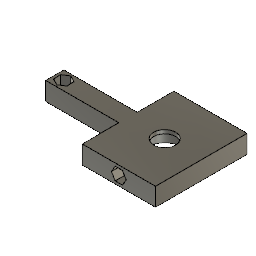
Hub Adapter (Autodesk Fusion 360 design; units mm, degrees)
Autodesk Fusion 360 part; units mm, degrees
sketch "Top" plane through (0, 0, 0) normal (0, 0, 1) x (1, 0, 0)
  line L0 (0, 0) -> (40, 0)
  line L1 (40, 0) -> (40, 50)
  line L2 (40, 50) -> (0, 50)
  line L3 (0, 50) -> (0, 0)
  circle A0 centre (20, 25) radius 11.2
  circle A1 centre (20, 25) radius 6
  dimension "d6" = 40
  dimension "d7" = 50
  dimension "d11" = 22.4
  dimension "d12" = 25
  dimension "d13" = 20
  dimension "d27" = 12
  constraint horizontal L0
  constraint vertical L1
  constraint horizontal L2
  constraint vertical L3
  constraint coincident L0.start L3.end
  constraint concentric A0 A1
  measures "d6" distance of L0.start L0.end
  measures "d7" distance of L0.start L2.end
  measures "d11" diameter of A0
  measures "d12" distance of L2 A0.centre
  measures "d13" distance of L1 A0.centre
  measures "d27" diameter of A1
extrude "Extrude1" add sketch "Top" along normal blind 10 contours L0 L1 L2 L3 | A0 | A1
extrude "Extrude2" cut sketch "Top" along normal blind 8 contours A0 | A1
extrude "Extrude5" cut sketch "Top" along normal blind 110 contours A1
sketch "Sketch3" plane through (0, 0, 0) normal (0, -1, 0) x (1, 0, 0)
  line L0 (0, 0) -> (40, 0)
  line L1 (40, 0) -> (40, 10)
  line L2 (40, 10) -> (0, 10)
  line L3 (0, 10) -> (0, 0)
  line L4 (24, 5) -> (22, 8.4641)
  line L5 (22, 8.4641) -> (18, 8.4641)
  line L6 (18, 8.4641) -> (16, 5)
  line L7 (16, 5) -> (18, 1.5359)
  line L8 (18, 1.5359) -> (22, 1.5359)
  line L9 (22, 1.5359) -> (24, 5)
  point P0 (20, 5)
  dimension "d34" = 4
  dimension "d37" = 20
  dimension "d38" = 5
  measures "d34" distance of L4.start P0
  measures "d37" distance of L3 P0
  measures "d38" distance of L2 P0
extrude "Extrude6" cut sketch "Sketch3" against normal blind 5 contours L4 L5 L6 L7 L8 L9
sketch "Sketch4" plane through (0, 50, 0) normal (0, 1, 0) x (-1, 0, 0)
  line L0 (-40, 0) -> (0, 0)
  line L1 (0, 0) -> (0, 10)
  line L2 (0, 10) -> (-40, 10)
  line L3 (-40, 10) -> (-40, 0)
  line L4 (-22.8284, 7.8284) -> (-23.8637, 3.9647)
  line L5 (-23.8637, 3.9647) -> (-21.0353, 1.1363)
  line L6 (-21.0353, 1.1363) -> (-17.1716, 2.1716)
  line L7 (-17.1716, 2.1716) -> (-16.1363, 6.0353)
  line L8 (-16.1363, 6.0353) -> (-18.9647, 8.8637)
  line L9 (-18.9647, 8.8637) -> (-22.8284, 7.8284)
  point P0 (-20, 5)
  dimension "d39" = 4
  dimension "d42" = 20
  dimension "d43" = 5
  measures "d39" distance of L4.start P0
  measures "d42" distance of L3 P0
  measures "d43" distance of L2 P0
extrude "Extrude7" cut sketch "Sketch4" against normal blind 5 contours L4 L5 L6 L7 L8 L9
sketch "Sketch5" plane through (0, 0, 0) normal (-1, 0, 0) x (0, -1, 0)
  line L0 (-50, 0) -> (0, 0)
  line L1 (0, 0) -> (0, 10)
  line L2 (0, 10) -> (-50, 10)
  line L3 (-50, 10) -> (-50, 0)
  line L4 (-30, 10) -> (-20, 10)
  line L5 (-20, 10) -> (-20, 0)
  line L6 (-20, 0) -> (-30, 0)
  line L7 (-30, 0) -> (-30, 10)
  dimension "d50" = 10
  dimension "d51" = 10
  dimension "d52" = 20
  constraint horizontal L4
  constraint vertical L5
  constraint horizontal L6
  constraint vertical L7
  constraint coincident L2 L4.start
  measures "d50" distance of L4.start L4.end
  measures "d51" distance of L4.start L6.end
  measures "d52" distance of L3 L7
extrude "Extrude8" add sketch "Sketch5" along normal blind 40 contours L0 L2 L4 L5 L6 L7
sketch "Sketch6" plane through (0, 0, 0) normal (0, 0, -1) x (1, 0, 0)
  circle A0 centre (20, -25) radius 11.2
  line L0 (0, -30) -> (0, -50)
  line L1 (0, -50) -> (40, -50)
  line L2 (40, -50) -> (40, 0)
  line L3 (40, 0) -> (0, 0)
  line L4 (0, 0) -> (0, -20)
  line L5 (0, -20) -> (-40, -20)
  line L6 (-40, -20) -> (-40, -30)
  line L7 (-40, -30) -> (0, -30)
  line L8 (-31.6559, -27.1948) -> (-31.4272, -23.2013)
  line L9 (-31.4272, -23.2013) -> (-34.7713, -21.0065)
  line L10 (-34.7713, -21.0065) -> (-38.3441, -22.8052)
  line L11 (-38.3441, -22.8052) -> (-38.5728, -26.7987)
  line L12 (-38.5728, -26.7987) -> (-35.2287, -28.9935)
  line L13 (-35.2287, -28.9935) -> (-31.6559, -27.1948)
  point P0 (-35, -25)
  dimension "d55" = 4
  dimension "d56" = 5
  dimension "d57" = 5
  measures "d55" distance of L8.start P0
  measures "d56" distance of L6 P0
  measures "d57" distance of L7 P0
extrude "Extrude9" cut sketch "Sketch6" against normal blind 100 contours L8 L9 L10 L11 L12 L13
equation "length = 50 mm"
equation "width = 40 mm"
equation "thickness = 10 mm"
equation "extra = 100 mm"
equation "fit_gap = 0.2 mm"
equation "d6 = width"
equation "d7 = length"
equation "d8 = thickness"
equation "bearing_outer_radius = 11.1 mm"
equation "d11 = ( bearing_outer_radius * 2 ) + fit_gap"
equation "d12 = length / 2"
equation "d13 = width / 2"
equation "d14 = thickness - 2 mm"
equation "bearing_inner_radius = ( 8 mm + 4 mm ) / 2"
equation "d27 = bearing_inner_radius * 2"
equation "d28 = thickness + extra"
equation "polygon_dowel_hole_side_length = 4 mm"
equation "polygon_dowel_hole_side_height = 5 mm"
equation "polygon_dowel_hole_big_distance = width / 2"
equation "polygon_dowel_hole_small_distance = thickness / 2"
equation "d34 = polygon_dowel_hole_side_length"
equation "d35 = -polygon_dowel_hole_side_height"
equation "d37 = polygon_dowel_hole_big_distance"
equation "d38 = polygon_dowel_hole_small_distance"
equation "d39 = polygon_dowel_hole_side_length"
equation "d40 = -polygon_dowel_hole_side_height"
equation "d42 = polygon_dowel_hole_big_distance"
equation "d43 = polygon_dowel_hole_small_distance"
equation "ackerman_bracket_length = 40 mm"
equation "ackerman_bracket_width = 10 mm"
equation "ackerman_bracket_big_distance = ( length - ackerman_bracket_width ) / 2"
equation "d50 = ackerman_bracket_width"
equation "d51 = ackerman_bracket_width"
equation "d52 = ackerman_bracket_big_distance"
equation "d53 = ackerman_bracket_length"
equation "d55 = polygon_dowel_hole_side_length"
equation "d56 = polygon_dowel_hole_small_distance"
equation "d57 = polygon_dowel_hole_small_distance"
equation "d58 = -extra"
